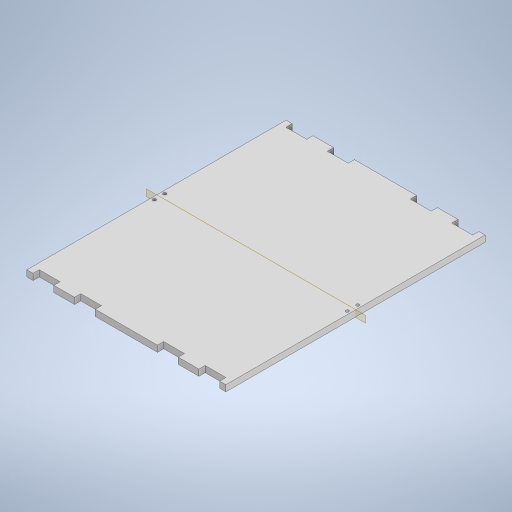
# Autodesk Inventor part: дно_пробитое
Saved by Autodesk Inventor 2024.2 (Build 282272000, 272)
## iProperties
Created: 2025-11-21
Part Number: дно_пробитое
Material: Типовые
Document SubType Name: Modeling
Designer: Zakhar
Density: 1 g/cm^3
Appearance: По умолчанию
Author: Zakhar
Autodesk Inventor part; units mm, degrees
ref_plane "YZ Plane" through (0, 0, 0) normal (1, 0, 0) x (0, 1, 0)
ref_plane "XZ Plane" through (0, 0, 0) normal (0, 1, 0) x (-1, 0, 0)
ref_plane "XY Plane" through (0, 0, 0) normal (0, 0, 1) x (1, 0, 0)
sketch "Эскиз1" plane through (0, 0, 0) normal (0, 1, 0) x (-1, 0, 0)
  line L0 (0, 250) -> (192, 250)
  line L1 (192, 250) -> (192, 0)
  line L2 (192, 0) -> (0, 0)
  line L3 (0, 0) -> (0, 250)
  circle A0 centre (11, 247) radius 1.5
  circle A1 centre (181, 247) radius 1.5
  circle A2 centre (5, 3) radius 1.5
  circle A3 centre (187, 3) radius 1.5
  line L4 (186, 6) -> (6, 6)
  line L5 (6, 6) -> (6, 244)
  line L6 (6, 244) -> (186, 244)
  line L7 (186, 244) -> (186, 6)
  dimension "d0" = 192
  dimension "d1" = 170
  dimension "d2" = 250
  dimension "d3" = 11
  dimension "d4" = 3
  dimension "d5" = 3
  dimension "d6" = 3
  dimension "d7" = 3
  dimension "d8" = 3
  dimension "d9" = 5
  dimension "d10" = 3
  dimension "d11" = 3
  dimension "d12" = 5
  dimension "d13" = 3
  dimension "d16" = 238
  dimension "d18" = 180
  dimension "d19" = 6
  dimension "d20" = 6
  constraints: 16 end point, 4 centre point, 4 parallel, 2 horizontal, 2 perpendicular, 1 coincident
  measures "d0" distance of L0.start L0.end
  measures "d1" distance of A0.centre A1.centre
  measures "d2" distance of L2.end L0.start
  measures "d3" distance from line of L3 A0.centre
  measures "d4" diameter of A0
  measures "d5" distance from line of L0 A0.centre
  measures "d6" distance from line of L0 A1.centre
  measures "d7" diameter of A1
  measures "d8" diameter of A2
  measures "d9" distance from line of A2.centre L3
  measures "d10" distance from line of L2 A2.centre
  measures "d11" diameter of A3
  measures "d12" distance from line of L1 A3.centre
  measures "d13" distance from line of L2 A3.centre
  measures "d16" distance of L4.end L5.end
  measures "d18" distance of L4.start L4.end
  measures "d19" distance between parallel lines of L2 L4
  measures "d20" distance between parallel lines of L3 L5
extrude "Выдавливание2" add sketch "Эскиз1" along normal blind 6 contours L0 L1 L2 L3 | A0 | A1 | A2 | A3 | L4 L5 L6 L7
sketch "Эскиз2" plane through (0, 0, 0) normal (0, -1, 0) x (1, 0, 0)
  line L0 (-192, 250) -> (0, 250) projected
  line L1 (-6, 250) -> (-26, 250)
  line L2 (-26, 250) -> (-26, 244)
  line L3 (-26, 244) -> (-6, 244)
  line L4 (-6, 244) -> (-6, 250)
  line L5 (-46, 250) -> (-66, 250)
  line L6 (-66, 250) -> (-66, 244)
  line L7 (-66, 244) -> (-46, 244)
  line L8 (-46, 244) -> (-46, 250)
  line L9 (-186, 250) -> (-166, 250)
  line L10 (-166, 250) -> (-166, 244)
  line L11 (-166, 244) -> (-186, 244)
  line L12 (-186, 244) -> (-186, 250)
  line L13 (-146, 250) -> (-126, 250)
  line L14 (-126, 250) -> (-126, 244)
  line L15 (-126, 244) -> (-146, 244)
  line L16 (-146, 244) -> (-146, 250)
  line L17 (0, 250) -> (0, 0) projected
  line L18 (-192, 0) -> (-192, 250) projected
  point P0 (-66, 247)
  point P1 (-46, 247)
  point P2 (-26, 247)
  point P3 (-146, 247)
  point P4 (-126, 247)
  point P5 (-166, 247)
  point P6 (-186, 247)
  dimension "d23" = 6
  dimension "d24" = 20
  dimension "d25" = 6
  dimension "d26" = 20
  dimension "d27" = 20
  dimension "d28" = 20
  dimension "d29" = 20
  dimension "d30" = 20
  dimension "d31" = 6
  constraints: 32 end point, 8 parallel, 7 midpoint, 7 point on line, 4 horizontal, 4 perpendicular
  measures "d23" distance between parallel lines of L4 L17
  measures "d24" distance of L2.end L3.end
  measures "d25" distance between parallel lines of L1 L3
  measures "d26" distance from line of point (-66, 247) L8
  measures "d27" distance of point (-46, 247) point (-26, 247)
  measures "d28" distance of point (-146, 247) point (-126, 247)
  measures "d29" distance of point (-166, 247) point (-146, 247)
  measures "d30" distance of point (-186, 247) point (-166, 247)
  measures "d31" distance from line of L18 point (-186, 247)
extrude "Выдавливание3" cut sketch "Эскиз2" against normal through all
ref_plane "РабПлоскость1" through (-126, 0, 125) normal (0, 0, 1) x (1, 0, 0)
mirror "Зеркальное отражение1" about plane through (-126, 0, 125) normal (0, 0, 1) of "Выдавливание3"
sketch "Эскиз3" plane through (0, 0, 0) normal (0, -1, 0) x (1, 0, 0)
  circle A0 centre (-3, 120) radius 1.5
  circle A1 centre (-3, 130) radius 1.5
  circle A2 centre (-189, 120) radius 1.5
  circle A3 centre (-189, 130) radius 1.5
  line L0 (-192, 0) -> (-192, 250) projected
  line L1 (-230.4, 125) -> (38.4, 125) projected
  line L2 (0, 250) -> (0, 0) projected
  dimension "d34" = 3
  dimension "d35" = 3
  dimension "d36" = 3
  dimension "d37" = 5
  dimension "d38" = 3
  dimension "d39" = 5
  dimension "d40" = 3
  dimension "d41" = 3
  dimension "d43" = 5
  dimension "d44" = 3
  dimension "d45" = 3
  dimension "d46" = 5
  constraints: 4 centre point
  measures "d34" diameter of A3
  measures "d35" diameter of A2
  measures "d36" distance from line of L0 A3.centre
  measures "d37" distance from line of L1 A3.centre
  measures "d38" distance from line of L0 A2.centre
  measures "d39" distance from line of L1 A2.centre
  measures "d40" distance from line of L2 A1.centre
  measures "d41" diameter of A1
  measures "d43" distance from line of L1 A1.centre
  measures "d44" diameter of A0
  measures "d45" distance from line of L2 A0.centre
  measures "d46" distance from line of L1 A0.centre
extrude "Выдавливание4" cut sketch "Эскиз3" against normal blind 10
equation "\"d26\" = d24"
equation "\"d27\" = d24"
equation "\"d28\" = d24"
equation "\"d29\" = d24"
equation "\"d30\" = d24"
